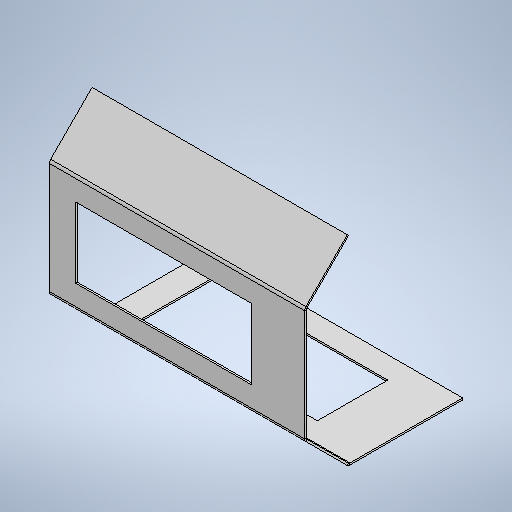
# Autodesk Inventor part: TKS 3554 BOTTOM DS box wall 1
Saved by Autodesk Inventor 2025 (Build 290162010, 162A)
## iProperties
Created: 2024-12-09
Part Number: TKS 3554 BOTTOM DS box wall 1
Material: Stainless Steel
Document SubType Name: Sheet Metal
Designer: user
Mass: 3269.02 g
Surface Area: 1007.63 cm^2
Volume: 408.627 cm^3
Density: 8 g/cm^3
Flat Pattern Width: 39.5348 cm
Flat Pattern Length: 29 cm
Flat Pattern Area: 1146.51 cm^2
Sheet Metal Rule: AISI304 2mm Die16
Sheet Metal Width: 395,348 mm
Sheet Metal Length: 290,000 mm
Sheet Metal Area: 114650,891 mm^2
Appearance: Default
Author: user
Autodesk Inventor part; units mm, degrees
ref_plane "YZ Plane" through (0, 0, 0) normal (1, 0, 0) x (0, 1, 0)
ref_plane "XZ Plane" through (0, 0, 0) normal (0, 1, 0) x (-1, 0, 0)
ref_plane "XY Plane" through (0, 0, 0) normal (0, 0, 1) x (1, 0, 0)
sketch "Sketch1" plane through (0, 0, 0) normal (0, 0, 1) x (1, 0, 0)
  line L0 (145, 65) -> (-145, 65)
  line L1 (-145, 65) -> (-145, -65)
  line L2 (-145, -65) -> (145, -65)
  line L3 (145, -65) -> (145, 65)
  line L4 (145, 65) -> (-145, -65) construction
  line L5 (-145, 65) -> (145, -65) construction
  line L6 (85, 40) -> (-115, 40)
  line L7 (-115, 40) -> (-115, -40)
  line L8 (-115, -40) -> (85, -40)
  line L9 (85, -40) -> (85, 40)
  line L10 (85, 40) -> (-115, -40) construction
  line L11 (-115, 40) -> (85, -40) construction
  point P0 (0, 0)
  point P1 (0, 0)
  point P2 (-15, 0)
  point P3 (85, 0)
  point P4 (145, 0)
  dimension "d34" = 200
  dimension "d35" = 80
  dimension "d51" = 60
  dimension "d53" = 30
  dimension "d54" = 25
  dimension "d56" = 130
  measures "d34" distance of L7.end L8.end
  measures "d35" distance of L8.end L6.start
  measures "d51" distance between parallel lines of L9 L3
  measures "d53" distance between parallel lines of L1 L7
  measures "d54" distance between parallel lines of L8 L2
  measures "d56" distance of L0.start L2.end
extrude "Plate1" add sketch "Sketch1" along normal blind 2
sketch "Sketch6" plane through (145, -63.5858, 1.4142) normal (0, -0.7071068, -0.7071068) x (1, 0, 0)
  line L0 (-290, 0) -> (0, 0)
  line L1 (0, 0) -> (0, 70)
  line L2 (0, 70) -> (-290, 70)
  line L3 (-290, 70) -> (-290, 0)
  constraints: 6 end point, 1 horizontal, 1 perpendicular, 1 vertical
edge flange "Flange2" height 70 angle 45 thickness 2 bend radius 2.75 thickness toward (0, -0.7071068, -0.7071068) relief round relief width 2 relief depth 1 edges at (0, -65, 2) wall of the first edge with corners at (-145, -63.5858, 1.4142) (145, -63.5858, 1.4142) (145, -113.0833, 50.9117) (-145, -113.0833, 50.9117)
bend "Bend2"
corner "Corner2"
sketch "Sketch8" plane through (145, -112.4975, 49.4975) normal (0, -1, 0) x (1, 0, 0)
  line L0 (-290, 0) -> (0, 0)
  line L1 (0, 0) -> (0, 130)
  line L2 (0, 130) -> (-290, 130)
  line L3 (-290, 130) -> (-290, 0)
  constraints: 6 end point, 1 horizontal, 1 perpendicular, 1 vertical
edge flange "Flange3" height 130 angle 45 thickness 2 bend radius 2.75 thickness toward (0, -1, 0) relief round relief width 2 relief depth 1 edges at (0, -113.0833, 50.9117) wall of the first edge with corners at (-145, -112.4975, 49.4975) (145, -112.4975, 49.4975) (145, -112.4975, 179.4975) (-145, -112.4975, 179.4975)
bend "Bend3"
corner "Corner3"
sketch "Sketch9" plane through (145, -113.0833, 178.0833) normal (0, -0.7071068, 0.7071068) x (1, 0, 0)
  line L0 (-290, 0) -> (0, 0)
  line L1 (0, 0) -> (0, 68.6)
  line L2 (0, 68.6) -> (-290, 68.6)
  line L3 (-290, 68.6) -> (-290, 0)
  constraints: 6 end point, 1 horizontal, 1 perpendicular, 1 vertical
edge flange "Flange4" height 68.6 angle 45 thickness 2 bend radius 2.75 thickness toward (0, -0.7071068, 0.7071068) relief round relief width 2 relief depth 1 edges at (0, -112.4975, 179.4975) wall of the first edge with corners at (-145, -113.0833, 178.0833) (145, -113.0833, 178.0833) (145, -64.5757, 226.5908) (-145, -64.5757, 226.5908)
bend "Bend4"
corner "Corner4"
sketch "Sketch10" plane through (-145, -114.4975, 51.465) normal (0, -1, 0) x (1, 0, 0)
  line L0 (290, 126.065) -> (0, 126.065) projected
  line L1 (0, 0) -> (0, 126.065) projected
  line L2 (0, 0) -> (290, 0) projected
  line L3 (290, 126.065) -> (290, 0) projected
  line L4 (30, 23.0325) -> (230, 23.0325)
  line L5 (230, 23.0325) -> (230, 103.0325)
  line L6 (230, 103.0325) -> (30, 103.0325)
  line L7 (30, 103.0325) -> (30, 23.0325)
  point P0 (145, -51.465)
  point P1 (30, 63.0325)
  point P2 (0, 63.0325)
  dimension "d77" = 80
  dimension "d78" = 200
  dimension "d79" = 30
  constraints: 8 end point, 2 midpoint, 2 parallel, 1 horizontal, 1 horizontal alignment, 1 perpendicular
  measures "d77" distance of L6.end L4.start
  measures "d78" distance of L5.end L6.end
  measures "d79" distance between parallel lines of L7 L1
extrude "Cut3" cut sketch "Sketch10" against normal blind 2 contours L7 L6 L5 L4
equation "\"d34\" = MAIN_6_central_window_hight"
equation "\"d35\" = MAIN_7_central_window_width"
equation "\"d56\" = Wall_1_width"
equation "\"d77\" = MAIN_7_central_window_width"
equation "\"d78\" = MAIN_6_central_window_hight"
equation "\"d79\" = d53"
equation "\"d80\" = Thickness"
equation "\"d2\" = Thickness"
equation "\"d36\" = BendReliefWidth"
equation "\"d37\" = BendReliefDepth"
equation "\"d38\" = MinimumRemnant"
equation "\"d39\" = TransitionRadius"
equation "\"d40\" = Wall_2_width"
equation "\"d42\" = BendRadius"
equation "\"d43\" = CornerReliefSize"
equation "\"d44\" = GapSize"
equation "\"d45\" = JacobiRadiusSize"
equation "\"d57\" = BendReliefWidth"
equation "\"d58\" = BendReliefDepth"
equation "\"d59\" = MinimumRemnant"
equation "\"d60\" = TransitionRadius"
equation "\"d61\" = d56"
equation "\"d63\" = BendRadius"
equation "\"d64\" = CornerReliefSize"
equation "\"d65\" = GapSize"
equation "\"d66\" = JacobiRadiusSize"
equation "\"d67\" = BendReliefWidth"
equation "\"d68\" = BendReliefDepth"
equation "\"d69\" = MinimumRemnant"
equation "\"d70\" = TransitionRadius"
equation "\"d71\" = Wall_2_width - 0.7 * Thickness"
equation "\"d73\" = BendRadius"
equation "\"d74\" = CornerReliefSize"
equation "\"d75\" = GapSize"
equation "\"d76\" = JacobiRadiusSize"
equation "\"BendReliefWidth\" = Thickness"
equation "\"BendReliefDepth\" = 0.5 * Thickness"
equation "\"CornerReliefSize\" = 4 * Thickness"
equation "\"MinimumRemnant\" = 2 * Thickness"
equation "\"TransitionRadius\" = BendRadius"
equation "\"JacobiRadiusSize\" = BendRadius"
equation "\"GapSize\" = Thickness"
equation "\"MAIN_6_central_window_hight\" = 200"
equation "\"MAIN_7_central_window_width\" = 80"
equation "\"Wall_1_width\" = 130"
equation "\"Thickness\" = 2"
equation "\"Wall_2_width\" = 70"
equation "\"BendRadius\" = 2.75"
body "Solid1"
